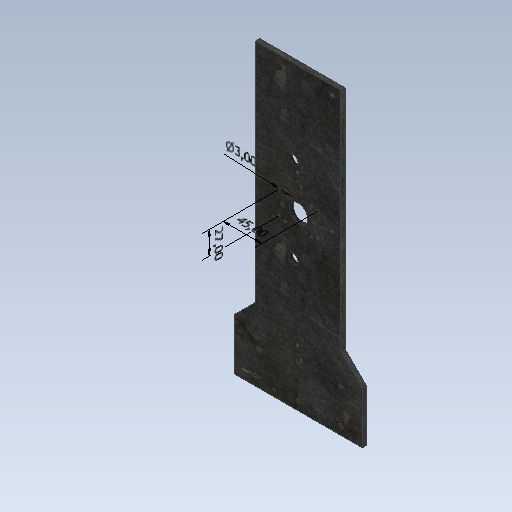
# Autodesk Inventor part: PlanchaLateral
Saved by Autodesk Inventor 2021 (Build 250183000, 183)
## iProperties
Created: 2022-05-28
Part Number: PlanchaLateral
Material: Acero ASTM A36
Document SubType Name: Modeling
Designer: 79449
Density: 7.85 g/cm^3
Appearance: Placa
Author: 79449
Autodesk Inventor part; units mm, degrees
ref_plane "YZ Plane" through (0, 0, 0) normal (1, 0, 0) x (0, 1, 0)
ref_plane "XZ Plane" through (0, 0, 0) normal (0, 1, 0) x (-1, 0, 0)
ref_plane "XY Plane" through (0, 0, 0) normal (0, 0, 1) x (1, 0, 0)
sketch "Boceto1" plane through (0, 0, 0) normal (0, 0, 1) x (1, 0, 0)
  line L0 (-75, 125) -> (75, 125) construction
  line L1 (75, 125) -> (75, -125) construction
  line L2 (75, -125) -> (-75, -125) construction
  line L3 (-75, -125) -> (-75, 125) construction
  line L4 (-75, 125) -> (75, -125) construction
  line L5 (75, 125) -> (-75, -125) construction
  line L6 (-75, -125) -> (75, -125)
  line L7 (75, -125) -> (75, -65)
  line L8 (-75, -125) -> (-75, -65)
  line L9 (-75, -65) -> (75, -65) construction
  line L10 (75, -65) -> (50, -40)
  line L11 (50, -40) -> (50, 125)
  line L12 (50, 125) -> (0, 125) construction
  line L13 (0, 125) -> (0, -125) construction
  line L14 (-75, -65) -> (-50, -40)
  line L15 (-50, -40) -> (-50, 125)
  line L16 (-50, 125) -> (0, 125) construction
  line L17 (-50, -40) -> (50, -40)
  circle A0 centre (0, 75) radius 11
  circle A1 centre (-22.5, 88.5) radius 1.5
  circle A2 centre (-22.5, 61.5) radius 1.5
  line L18 (-22.5, 88.5) -> (-22.5, 61.5) construction
  line L19 (0, 75) -> (-22.5, 75) construction
  circle A3 centre (22.5, 88.5) radius 1.5
  circle A4 centre (22.5, 61.5) radius 1.5
  circle A5 centre (-6, 26) radius 6
  line L20 (-75, -115) -> (75, -115) construction
  line L21 (-75, -75) -> (75, -75) construction
  circle A6 centre (0, -75) radius 2.5
  circle A7 centre (0, -115) radius 2.5
  circle A8 centre (50, -75) radius 2.5
  circle A9 centre (50, -115) radius 2.5
  circle A10 centre (-50, -75) radius 2.5
  circle A11 centre (-50, -115) radius 2.5
  line L22 (-50, 125) -> (50, 125) construction
  line L23 (50, 125) -> (50, 225)
  line L24 (50, 225) -> (-50, 225)
  line L25 (-50, 225) -> (-50, 125)
  line L26 (0, 225) -> (0, -40) construction
  circle A12 centre (-6, 126) radius 6
  circle A13 centre (18.5, 75) radius 2.5
  circle A14 centre (-18.5, 75) radius 2.5
  circle A15 centre (-15.5, 90.5) radius 1.5
  circle A16 centre (15.5, 90.5) radius 1.5
  line L27 (-15.5, 90.5) -> (15.5, 90.5) construction
  circle A17 centre (-15.5, 59.5) radius 1.5
  circle A18 centre (15.5, 59.5) radius 1.5
  circle A19 centre (-17, 215) radius 2.1
  circle A20 centre (40, 215) radius 2.1
  line L28 (-17, 215) -> (40, 215) construction
  circle A21 centre (40, 77.2) radius 2.1
  line L29 (40, 215) -> (40, 77.2) construction
  point P0 (0, 0)
  dimension "d0" = 150
  dimension "d1" = 250
  dimension "d2" = 60
  dimension "d3" = 45
  dimension "d4" = 50
  dimension "d6" = 22
  dimension "d8" = 3
  dimension "d9" = 3
  dimension "d10" = 27
  dimension "d11" = 22.5
  dimension "d16" = 10
  dimension "d17" = 40
  dimension "d18" = 5
  dimension "d19" = 5
  dimension "d20" = 5
  dimension "d21" = 5
  dimension "d22" = 50
  dimension "d23" = 50
  dimension "d25" = 12
  dimension "d29" = 100
  dimension "d30" = 6
  dimension "d31" = 115
  dimension "d32" = 66
  dimension "d34" = 6
  dimension "d35" = 166
  dimension "d36" = 12
  dimension "d48" = 13.5
  dimension "d49" = 18.5
  dimension "d50" = 5
  dimension "d52" = 15.5
  dimension "d53" = 15.5
  dimension "d54" = 15.5
  dimension "d55" = 3
  dimension "d56" = 3
  dimension "d57" = 10
  dimension "d59" = 4.2
  dimension "d60" = 4.2
  dimension "d61" = 57
  dimension "d63" = 4.2
  dimension "d64" = 10
  dimension "d65" = 137.8
  constraints: 60 end point, 22 centre point, 11 point on line, 9 midpoint, 9 symmetric about line, 6 perpendicular, 5 horizontal, 4 parallel, 2 collinear, 2 vertical, 7 other
  measures "d0" distance of L0.start L0.end
  measures "d1" distance of L0.end L1.end
  measures "d2" distance of L7.end L1.end
  measures "d3" angle of L10 L9
  measures "d4" horizontal distance of point (0, 0) L10.end
  measures "d6" diameter of A0
  measures "d8" diameter of A2
  measures "d9" diameter of A1
  measures "d10" distance of L18.end L18.start
  measures "d11" distance from line of L19.start L18
  measures "d16" distance between parallel lines of L20 L2
  measures "d17" distance between parallel lines of L21 L20
  measures "d18" diameter of A6
  measures "d19" diameter of A7
  measures "d20" diameter of A9
  measures "d21" diameter of A8
  measures "d22" distance of A6.centre A8.centre
  measures "d23" distance of A7.centre A9.centre
  measures "d25" diameter of A5
  measures "d29" distance between parallel lines of L0 L24
  measures "d30" distance from line of L13 A5.centre
  measures "d31" distance from line of L17 L19.start
  measures "d32" distance from line of L17 A5.centre
  measures "d34" distance from line of L26 A12.centre
  measures "d35" distance from line of L17 A12.centre
  measures "d36" diameter of A12
  measures "d48" distance from line of L18.end L19
  measures "d49" distance of L19.start A13.centre
  measures "d50" diameter of A13
  measures "d52" distance from line of L26 L27.end
  measures "d53" distance from line of L27.start L26
  measures "d54" distance from line of L27.start L19
  measures "d55" diameter of A15
  measures "d56" diameter of A16
  measures "d57" distance from line of L24 L28.start
  measures "d59" diameter of A19
  measures "d60" diameter of A20
  measures "d61" distance of L28.start L28.end
  measures "d63" diameter of A21
  measures "d64" distance from line of L23 L28.end
  measures "d65" distance of L28.end L29.end
extrude "Extrusión1" add sketch "Boceto1" along normal blind 5
